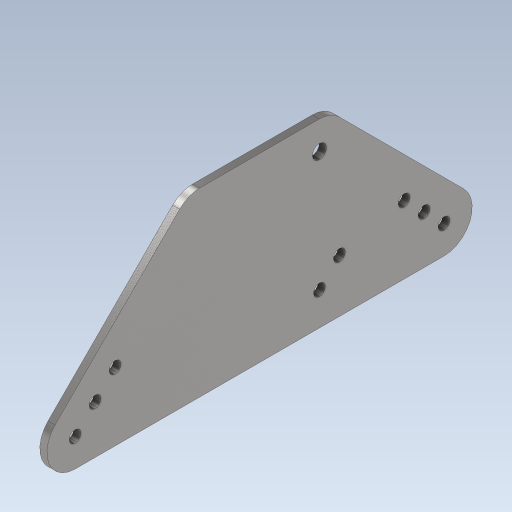
# Autodesk Inventor part: HipPivotPlate
Saved by Autodesk Inventor 2023 (Build 270158000, 158)
## iProperties
Created: 2023-04-06
Part Number: HipPivotPlate
Material: Aluminum 6061
Document SubType Name: Modeling
Designer: Dave
Density: 2.7 g/cm^3
Appearance: Galvanized
Mass: 96.5969 g
Surface Area: 244.776 cm^2
Volume: 35.7766 cm^3
Author: Dave
Autodesk Inventor part; units mm, degrees
ref_plane "YZ Plane" through (0, 0, 0) normal (1, 0, 0) x (0, 1, 0)
ref_plane "XZ Plane" through (0, 0, 0) normal (0, 1, 0) x (-1, 0, 0)
ref_plane "XY Plane" through (0, 0, 0) normal (0, 0, 1) x (1, 0, 0)
sketch "Sketch1" plane through (0, 0, 0) normal (1, 0, 0) x (0, 1, 0)
  circle A0 centre (0, 0) radius 3.175
  circle A1 centre (-56.0605, -56.0605) radius 2.65
  circle A2 centre (-38.1, -38.1) radius 2.65
  circle A3 centre (-47.0803, 100.9618) radius 2.65
  circle A4 centre (-56.0605, 109.942) radius 2.65
  circle A5 centre (-38.1, 91.9815) radius 2.65
  circle A6 centre (-47.0803, -47.0803) radius 2.65
  line L0 (-47.0803, 100.9618) -> (16.1666, 37.7149) construction
  line L1 (-38.1, -38.1) -> (-38.3774, -38.3774) construction
  line L2 (-28.0876, 28.0876) -> (0, 0) construction
  line L3 (0, 0) -> (-28.0876, -28.0876) construction
  line L4 (0, 0) -> (18.6115, 0) construction
  line L5 (-47.0803, 118.9223) -> (8.9803, 62.8618)
  line L6 (12.7, 53.8815) -> (12.7, 0)
  line L7 (-65.0408, -118.9223) -> (-65.0408, -118.9223)
  line L8 (-68.7605, -56.0605) -> (-68.7605, 109.942)
  line L9 (-65.0408, 118.9223) -> (-65.0408, 118.9223)
  arc A7 (12.7, 53.8815) -> (8.9803, 62.8618) centre (0, 53.8815) ccw
  arc A8 (-65.0408, 118.9223) -> (-68.7605, 109.942) centre (-56.0605, 109.942) ccw
  arc A9 (-47.0803, 118.9223) -> (-65.0408, 118.9223) centre (-56.0605, 109.942) ccw
  line L10 (-47.0803, -65.0408) -> (8.9803, -8.9803)
  arc A10 (8.9803, -8.9803) -> (12.7, 0) centre (0, 0) ccw
  arc A11 (-68.7605, -56.0605) -> (-47.0803, -65.0408) centre (-56.0605, -56.0605) ccw
  line L11 (-26.9408, -8.9802) -> (-44.9013, -26.9407) projected
  line L12 (-44.9013, -26.9407) -> (-284.0015, 212.1595) projected
  line L13 (-266.041, 230.12) -> (-284.0015, 212.1595) projected
  line L14 (-26.9408, -8.9802) -> (-266.041, 230.12) projected
  circle A12 centre (-53.8816, 0) radius 2.65
  circle A13 centre (-44.9013, -8.9802) radius 2.65
  line L15 (-53.8816, 0) -> (-44.9013, -8.9802) construction
  circle A14 centre (-100, 0) radius 12.3551
  point P0 (12.7, -5.2605)
  point P1 (-68.7605, -86.721)
  point P2 (-65.0408, 118.9223)
  dimension "d0" = 6.35
  dimension "d1" = 5.3
  dimension "d2" = 5.3
  dimension "d3" = 5.3
  dimension "d4" = 5.3
  dimension "d5" = 5.3
  dimension "d6" = 5.3
  dimension "d7" = 135
  dimension "d8" = 38.1
  dimension "d10" = 38.1
  dimension "d11" = 12.7
  dimension "d12" = 12.7
  dimension "d13" = 38.1
  dimension "d14" = 12.7
  dimension "d15" = 12.7
  dimension "d16" = 12.7
  dimension "d17" = 12.7
  dimension "d18" = 12.7
  dimension "d19" = 45
  dimension "d20" = 12.7
  dimension "d21" = 12.7
  dimension "d24" = 12.7
  dimension "d25" = 12.7
  dimension "d26" = 12.7
  dimension "d27" = 12.7
  dimension "d29" = 12.7
  dimension "d30" = 100
  constraints: 24 end point, 15 centre point, 10 point on circle, 10 tangent, 8 point on line, 5 equal radius, 4 parallel, 3 perpendicular, 2 collinear, 1 coincident, 1 horizontal, 1 vertical, 1 other
  measures "d0" diameter of A0
  measures "d1" diameter of A1
  measures "d2" diameter of A2
  measures "d3" diameter of A3
  measures "d4" diameter of A4
  measures "d5" diameter of A5
  measures "d6" diameter of A6
  measures "d7" angle of L4 L3
  measures "d8" distance between parallel lines of L2 L0
  measures "d10" horizontal distance of A5.centre point (0, 0)
  measures "d11" distance of A5.centre L0.start
  measures "d12" distance of L0.start A4.centre
  measures "d13" horizontal distance of L1.start point (0, 0)
  measures "d14" distance of A6.centre L1.start
  measures "d15" distance of A1.centre A6.centre
  measures "d16" distance from line of L5 A5.centre
  measures "d17" distance from line of L9 A4.centre
  measures "d18" distance from line of L6 point (0, 0)
  measures "d19" angle of L6 L5
  measures "d20" distance from line of L8 A4.centre
  measures "d21" radius of A7
  measures "d24" radius of A10
  measures "d25" distance from line of L10 A1.centre
  measures "d26" distance of L15.start L15.end
  measures "d27" distance between parallel lines of L14 L15
  measures "d29" distance from line of L11 L15.end
  measures "d30" distance of A14.centre point (0, 0)
extrude "Extrusion1" add sketch "Sketch1" along normal blind 3.175 contours L5 A7 L6 A10 L10 A11 L8 L12 L11 L14 A8 A9 | L14 L11 L12 L8
equation "\"d12\" = d11"
equation "\"d13\" = d10"
equation "\"d14\" = d11"
equation "\"d15\" = d11"
body "Solid1"
